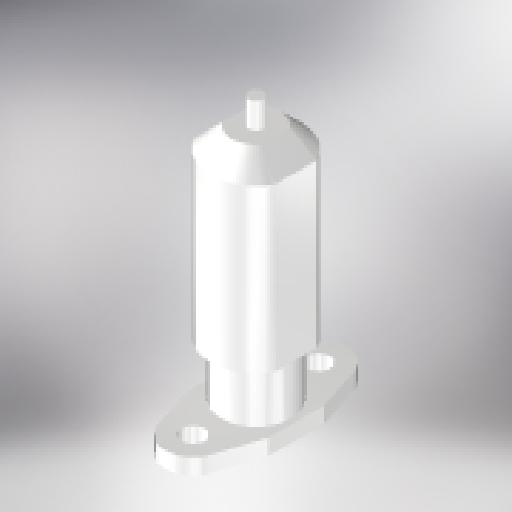
# Autodesk Inventor part: BLTouch
Saved by Autodesk Inventor 2023 (Build 270158000, 158)
## iProperties
Created: 2022-06-28
Part Number: BLTouch
Material: ABS Plastic
Document SubType Name: Modeling
Designer: Remo
Density: 1.06 g/cm^3
Appearance: Smooth - White
Author: Remo
Autodesk Inventor part; units mm, degrees
ref_plane "YZ Plane" through (0, 0, 0) normal (1, 0, 0) x (0, 1, 0)
ref_plane "XZ Plane" through (0, 0, 0) normal (0, 1, 0) x (-1, 0, 0)
ref_plane "XY Plane" through (0, 0, 0) normal (0, 0, 1) x (1, 0, 0)
sketch "Sketch1" plane through (0, 0, 0) normal (0, 1, 0) x (-1, 0, 0)
  line L0 (-5.765, 13) -> (5.765, 13)
  line L1 (5.765, 13) -> (5.765, -13)
  line L2 (5.765, -13) -> (-5.765, -13)
  line L3 (-5.765, -13) -> (-5.765, 13)
  line L4 (-5.765, 13) -> (5.765, -13) construction
  line L5 (5.765, 13) -> (-5.765, -13) construction
  circle A0 centre (0, 9) radius 1.6
  circle A1 centre (0, -9) radius 1.6
  circle A2 centre (0, 9) radius 4
  circle A3 centre (0, -9) radius 4
  line L6 (5.765, 4) -> (3.8159, 10.1997)
  line L7 (3.8159, -10.1997) -> (5.765, -4)
  line L8 (-3.8159, -10.1997) -> (-5.765, -4)
  line L9 (-5.765, 4) -> (-3.8159, 10.1997)
  point P0 (0, 0)
  dimension "d0" = 26
  dimension "d1" = 11.53
  dimension "d2" = 18
  dimension "d3" = 9
  dimension "d4" = 3.2
  dimension "d5" = 8
  dimension "d6" = 4
  dimension "d7" = 4
  constraints: 20 end point, 4 centre point, 4 point on circle, 4 point on line, 4 tangent, 3 parallel, 2 coincident, 2 equal radius, 2 midpoint, 2 vertical alignment, 1 equal length, 1 horizontal, 1 perpendicular
  measures "d0" distance of L0.end L1.end
  measures "d1" distance between parallel lines of L3 L1
  measures "d2" distance of A1.centre A0.centre
  measures "d3" distance of point (0, 0) A1.centre
  measures "d4" diameter of A0
  measures "d5" diameter of A2
  measures "d6" vertical distance of L6.start point (0, 0)
  measures "d7" vertical distance of L7.end point (0, 0)
extrude "Extrusion1" add sketch "Sketch1" along normal blind 2.3 contours A2 | L9 A2 L6 L1 L7 A3 L8 L3 | A3
sketch "Sketch2" plane through (0, 2.3, 0) normal (0, 1, 0) x (1, 0, 0)
  line L0 (5.765, -4) -> (5.765, 4) projected
  line L1 (5.765, 4) -> (3.8159, 10.1997) projected
  arc A0 (3.8159, 10.1997) -> (-3.8159, 10.1997) centre (0, 9) ccw projected
  line L2 (-3.8159, 10.1997) -> (-5.765, 4) projected
  line L3 (-5.765, 4) -> (-5.765, -4) projected
  line L4 (-5.765, -4) -> (-3.8159, -10.1997) projected
  arc A1 (-3.8159, -10.1997) -> (3.8159, -10.1997) centre (0, -9) ccw projected
  line L5 (3.8159, -10.1997) -> (5.765, -4) projected
  circle A2 centre (0, -9) radius 1.6 projected
  circle A3 centre (0, 9) radius 1.6 projected
  circle A4 centre (0, 0) radius 5
  dimension "d10" = 10
  constraints: 1 centre point, 1 coincident
  measures "d10" diameter of A4
extrude "Extrusion2" add sketch "Sketch2" along normal blind 7.7 contours A4
sketch "Sketch3" plane through (0, 10, 0) normal (0, 1, 0) x (1, 0, 0)
  circle A0 centre (0, 0) radius 5 projected
  line L0 (5.765, 6.5) -> (-5.765, 6.5)
  line L1 (-5.765, 6.5) -> (-5.765, -6.5)
  line L2 (-5.765, -6.5) -> (5.765, -6.5)
  line L3 (5.765, -6.5) -> (5.765, 6.5)
  line L4 (5.765, 6.5) -> (-5.765, -6.5) construction
  line L5 (-5.765, 6.5) -> (5.765, -6.5) construction
  circle A1 centre (0, 0) radius 6.5
  point P0 (-5.765, 4)
  point P1 (5.765, -3.0025)
  point P2 (5.765, 3.0025)
  point P3 (-5.765, 3.0025)
  point P4 (-5.765, -3.0025)
  dimension "d13" = 13
  constraints: 12 end point, 2 midpoint, 2 parallel, 1 centre point, 1 coincident, 1 horizontal, 1 perpendicular, 1 tangent, 1 vertical alignment
  measures "d13" distance between parallel lines of L0 L2
extrude "Extrusion3" add sketch "Sketch3" along normal blind 26.3 contours A0 | A1 L3 L1
sketch "Sketch4" plane through (0, 36.3, 0) normal (0, 1, 0) x (1, 0, 0)
  circle A0 centre (0, 0) radius 1
  dimension "d19" = 2
  constraints: 1 centre point, 1 coincident
  measures "d19" diameter of A0
chamfer "Chamfer1" distance 3 angle 45 4 edges at (0, 36.3, -6.5) (0, 36.3, 6.5) (5.765, 36.3, 0) (-5.765, 36.3, 0)
extrude "Extrusion4" add sketch "Sketch4" along normal blind 3.7
equation "\"d3\" = 0.5 * d2"
equation "\"d7\" = d6"
body "Solid1"
